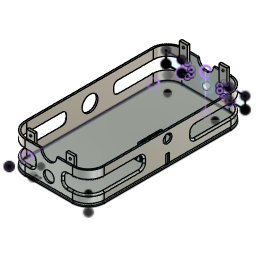
enclosure_bottom (Autodesk Fusion 360 design; units mm, degrees)
Autodesk Fusion 360 part; units mm, degrees
sketch "Sketch1" plane through (0, 0, 0) normal (0, 0, 1) x (1, 0, 0)
  line L0 (20, 0) -> (80, 0)
  line L1 (100, 20) -> (100, 180)
  line L2 (80, 200) -> (20, 200)
  line L3 (0, 180) -> (0, 20)
  arc A0 (0, 20) -> (20, 0) centre (20, 20) ccw
  arc A1 (80, 0) -> (100, 20) centre (80, 20) ccw
  arc A2 (100, 180) -> (80, 200) centre (80, 180) ccw
  arc A3 (20, 200) -> (0, 180) centre (20, 180) ccw
  line L4 (20, 2) -> (80, 2)
  arc A4 (80, 2) -> (98, 20) centre (80, 20) ccw
  line L5 (98, 20) -> (98, 180)
  arc A5 (98, 180) -> (80, 198) centre (80, 180) ccw
  line L6 (80, 198) -> (20, 198)
  arc A6 (20, 198) -> (2, 180) centre (20, 180) ccw
  line L7 (2, 180) -> (2, 20)
  arc A7 (2, 20) -> (20, 2) centre (20, 20) ccw
  point P0 (100, 0)
  point P1 (0, 200)
  dimension "d1" = 100
  dimension "d2" = 200
  dimension "d3" = 20
  dimension "d4" = -2
  constraint horizontal L0
  constraint vertical L1
  constraint horizontal L2
  constraint vertical L3
  constraint coincident origin L0
  constraint coincident origin L3
  constraint tangent L0 A0
  constraint tangent L3 A0
  constraint coincident P0 L0
  constraint coincident P0 L1
  constraint tangent L0 A1
  constraint tangent L1 A1
  constraint equal A0 A1
  constraint tangent L1 A2
  constraint tangent L2 A2
  constraint equal A0 A2
  constraint coincident P1 L2
  constraint coincident P1 L3
  constraint tangent L2 A3
  constraint tangent L3 A3
  constraint equal A0 A3
  measures "d1" distance of origin P0
  measures "d2" distance of origin P1
  measures "d3" radius of A0
extrude "Extrude1" add sketch "Sketch1" along normal blind 1.5 contours L4 A4 L5 A5 L6 A6 L7 A7
extrude "Extrude2" add sketch "Sketch1" along normal blind 40
sketch "Sketch2" plane through (0, 0, 0) normal (0, -1, 0) x (1, 0, 0)
  line L0 (20, 0) -> (80, 0)
  line L1 (80, 0) -> (80, 40)
  line L2 (80, 40) -> (20, 40)
  line L3 (20, 40) -> (20, 0)
  circle A0 centre (50, 40) radius 10
  dimension "d9" = 20
  constraint midpoint L2 A0.centre
  measures "d9" diameter of A0
sketch "Sketch3" plane through (0, 200, 0) normal (0, 1, 0) x (-1, 0, 0)
  line L0 (-80, 0) -> (-20, 0)
  line L1 (-20, 0) -> (-20, 40)
  line L2 (-20, 40) -> (-80, 40)
  line L3 (-80, 40) -> (-80, 0)
  circle A0 centre (-50, 40) radius 10
  dimension "d10" = 20
  constraint midpoint L2 A0.centre
  measures "d10" diameter of A0
extrude "Extrude3" cut sketch "Sketch3" against normal blind 10 contours L2 A0 picked at (-47.135, 36.6429)
extrude "Extrude4" cut sketch "Sketch2" against normal blind 10 contours L2 A0 picked at (52.865, 36.6429)
sketch "Sketch4" plane through (0, 0, 0) normal (-1, 0, 0) x (0, -1, 0)
  line L0 (-180, 0) -> (-20, 0)
  line L1 (-20, 0) -> (-20, 40)
  line L2 (-20, 40) -> (-180, 40)
  line L3 (-180, 40) -> (-180, 0)
  line L4 (-179.9999, 28) -> (-134.9999, 28)
  line L5 (-129.9999, 23) -> (-129.9999, 18)
  line L6 (-134.9999, 13) -> (-179.9999, 13)
  line L7 (-179.9999, 13) -> (-179.9999, 28)
  line L8 (-100, 40) -> (-100, 0) construction
  line L9 (-65.0001, 13) -> (-20.0001, 13)
  line L10 (-70.0001, 23) -> (-70.0001, 18)
  line L11 (-20.0001, 28) -> (-65.0001, 28)
  line L12 (-20.0001, 13) -> (-20.0001, 28)
  arc A0 (-129.9999, 23) -> (-134.9999, 28) centre (-134.9999, 23) ccw
  arc A1 (-134.9999, 13) -> (-129.9999, 18) centre (-134.9999, 18) ccw
  arc A2 (-65.0001, 28) -> (-70.0001, 23) centre (-65.0001, 23) ccw
  arc A3 (-70.0001, 18) -> (-65.0001, 13) centre (-65.0001, 18) ccw
  line L13 (-179.9999, 13) -> (-219.9999, 13)
  line L14 (-219.9999, 13) -> (-219.9999, 28)
  line L15 (-219.9999, 28) -> (-179.9999, 28)
  line L16 (-179.9999, 28) -> (-179.9999, 13)
  circle A4 centre (-100, 20) radius 10
  point P0 (-129.9999, 28)
  dimension "d15" = 50
  dimension "d16" = 15
  dimension "d17" = 0.0001
  dimension "d18" = 12
  dimension "d24" = 5
  dimension "d57" = 40
  dimension "d58" = 15
  dimension "d124" = 20
  dimension "d139" = 20
  constraint horizontal L4
  constraint vertical L5
  constraint horizontal L6
  constraint vertical L7
  constraint midpoint L2 L8.start
  constraint perpendicular L2 L8
  constraint symmetric L4.start L8 L11.start
  constraint symmetric L6.end L8 L9.end
  constraint coincident P0 L4
  constraint coincident P0 L5
  constraint tangent L4 A0
  constraint tangent L5 A0
  constraint tangent L5 A1
  constraint tangent L6 A1
  constraint equal A0 A1
  constraint tangent L10 A2
  constraint tangent L11 A2
  constraint equal A0 A2
  constraint tangent L9 A3
  constraint tangent L10 A3
  constraint equal A0 A3
  constraint horizontal L13
  constraint vertical L14
  constraint horizontal L15
  constraint vertical L16
  constraint midpoint L8 A4.centre
  measures "d15" distance of L4.start P0
  measures "d16" distance of L4.start L6.end
  measures "d17" distance of L3 L7
  measures "d18" distance of L2 L4
  measures "d24" radius of A0
  measures "d57" distance of L6.end L13.end
  measures "d58" distance of L6.end L4.start
  measures "d124" diameter of A4
  measures "d139" distance of L2 A4.centre
sketch "Sketch5" plane through (0, 0, 0) normal (0, -1, 0) x (1, 0, 0)
  arc A0 (40, 40) -> (60, 40) centre (50, 40) ccw
  line L0 (40, 40) -> (20, 40)
  line L1 (20, 40) -> (20, 0)
  line L2 (20, 0) -> (80, 0)
  line L3 (80, 0) -> (80, 40)
  line L4 (80, 40) -> (60, 40)
  line L5 (20, 28) -> (27, 28)
  line L6 (32, 23) -> (32, 18)
  line L7 (27, 13) -> (20, 13)
  line L8 (20, 13) -> (20, 28)
  line L9 (50, 30) -> (50, -15.7187) construction
  line L10 (50, 30) -> (50, -15.7187) construction
  line L11 (73, 13) -> (80, 13)
  line L12 (68, 23) -> (68, 18)
  line L13 (80, 28) -> (73, 28)
  line L14 (80, 13) -> (80, 28)
  line L15 (20, 28) -> (0, 28)
  line L16 (0, 28) -> (0, 13)
  line L17 (0, 13) -> (20, 13)
  line L18 (20, 13) -> (20, 28)
  line L19 (100, 13) -> (80, 13)
  line L20 (100, 28) -> (100, 13)
  line L21 (80, 28) -> (100, 28)
  line L22 (80, 13) -> (80, 28)
  arc A1 (32, 23) -> (27, 28) centre (27, 23) ccw
  arc A2 (27, 13) -> (32, 18) centre (27, 18) ccw
  arc A3 (68, 18) -> (73, 13) centre (73, 18) ccw
  arc A4 (73, 28) -> (68, 23) centre (73, 23) ccw
  arc A5 (20, 28) -> (20, 13) centre (20, 20.5) ccw
  line L23 (20, 13) -> (2, 13)
  line L24 (2, 28) -> (20, 28)
  circle A6 centre (50, 13.9414) radius 6.75
  point P0 (32, 28)
  dimension "d19" = 12
  dimension "d20" = 15
  dimension "d21" = 12
  dimension "d22" = 20
  dimension "d23" = 15
  dimension "d25" = 5
  dimension "d54" = 18
  dimension "d140" = 13.5
  constraint horizontal L5
  constraint vertical L6
  constraint horizontal L7
  constraint vertical L8
  constraint coincident L1 L5.start
  constraint midpoint A0 L9.start
  constraint vertical L9
  constraint symmetric L5.start L9 L13.start
  constraint symmetric L7.end L9 L11.end
  constraint symmetric L10.start L9 L9.start
  constraint symmetric L10.end L9 L9.end
  constraint horizontal L15
  constraint vertical L16
  constraint horizontal L17
  constraint vertical L18
  constraint symmetric L9 L15.end L20.start
  constraint symmetric L9 L16.end L19.start
  constraint symmetric L9 L7.end L11.end
  constraint coincident P0 L5
  constraint coincident P0 L6
  constraint tangent L5 A1
  constraint tangent L6 A1
  constraint tangent L6 A2
  constraint tangent L7 A2
  constraint equal A1 A2
  constraint tangent L11 A3
  constraint tangent L12 A3
  constraint equal A1 A3
  constraint tangent L12 A4
  constraint tangent L13 A4
  constraint equal A1 A4
  constraint tangent L5 A5
  constraint coincident L17 L23.end
  constraint coincident L15 L24.start
  constraint tangent A5 L24
  constraint coincident L9 A6.centre
  measures "d19" distance of L5.start P0
  measures "d20" distance of L5.start L7.end
  measures "d21" distance of L0 L5
  measures "d22" distance of L5.start L15.end
  measures "d23" distance of L5.start L7.end
  measures "d25" radius of A1
  measures "d54" distance of L7.end L23.end
  measures "d140" diameter of A6
extrude "Extrude5" cut sketch "Sketch5" against normal blind 21 contours L1 L5 L6 L7 L8 L18 A1 A2 | L15 L16 L17 A5 L23 L24 | L1 L8 L18 A5
extrude "Extrude6" cut sketch "Sketch4" against normal blind 10 contours L1 L9 L10 L11 L12 A2 A3
ref_plane "WorkPlane1" through (0, 100, 0) normal (0, 1, 0) x (0, 0, 1)
ref_plane "WorkPlane2" through (50, 0, 0) normal (1, 0, 0) x (0, 1, 0)
extrude "Extrude7" cut sketch "Sketch4" against normal blind 10 contours L3 L4 L5 L6 L7 A0 A1 L16
extrude "Extrude8" cut sketch "Sketch5" against normal blind 21 contours L3 L14 L19 L20 L21 L22 | L3 L11 L12 L13 L14 L22 A3 A4
sketch "Sketch6" plane through (0, 198, 0) normal (0, -1, 0) x (1, 0, 0)
  arc A0 (40, 40) -> (60, 40) centre (50, 40) ccw
  line L0 (40, 40) -> (20, 40)
  line L1 (20, 40) -> (20, 1.5)
  line L2 (20, 1.5) -> (80, 1.5)
  line L3 (80, 1.5) -> (80, 40)
  line L4 (80, 40) -> (60, 40)
  line L5 (80, 28) -> (100, 28)
  line L6 (80, 28) -> (73, 28)
  arc A1 (73, 28) -> (68, 23) centre (73, 23) ccw
  line L7 (68, 23) -> (68, 18)
  arc A2 (68, 18) -> (73, 13) centre (73, 18) ccw
  line L8 (73, 13) -> (80, 13)
  line L9 (100, 13) -> (80, 13)
  line L10 (32, 23) -> (32, 18)
  arc A3 (32, 23) -> (27, 28) centre (27, 23) ccw
  line L11 (20, 28) -> (27, 28)
  line L12 (20, 28) -> (0, 28)
  arc A4 (27, 13) -> (32, 18) centre (27, 18) ccw
  line L13 (27, 13) -> (20, 13)
  line L14 (0, 13) -> (20, 13)
  line L15 (0, 28) -> (0, 13)
  line L16 (100, 28) -> (100, 13)
  line L17 (0, 28) -> (0, 13)
  line L18 (100, 28) -> (80, 28)
  line L19 (80, 28) -> (80, 13)
  line L20 (80, 13) -> (100, 13)
  line L21 (20, 28) -> (0, 28)
  line L22 (0, 13) -> (20, 13)
  line L23 (50, 30) -> (50, -15.7187)
  line L24 (20, 13) -> (0, 13)
  line L25 (0, 28) -> (0, 13)
  line L26 (0, 28) -> (20, 28)
  line L27 (20, 28) -> (20, 13)
  constraint coincident L12.end L15.start
  constraint coincident L14.start L15.end
  constraint coincident L5.end L16.start
  constraint coincident L9.start L16.end
  constraint coincident L5.start L6.start
  constraint coincident L8.end L9.end
  constraint coincident L11.start L12.start
  constraint coincident L13.end L14.end
  constraint symmetric L5.end L23 L12.end
  constraint symmetric L9.start L23 L14.start
  constraint symmetric L5.start L23 L11.start
  constraint symmetric L8.end L23 L13.end
extrude "Extrude13" cut sketch "Sketch6" along normal blind 21 contours L3 L5 L9 L16 L18 L19 L20
sketch "Sketch7" plane through (100, 0, 0) normal (1, 0, 0) x (0, 1, 0)
  line L0 (20, 28) -> (21, 28)
  line L1 (21, 28) -> (21, 13)
  line L2 (21, 13) -> (20, 13)
  line L3 (20, 13) -> (20, 0)
  line L4 (20, 0) -> (180, 0)
  line L5 (180, 28) -> (180, 40)
  line L6 (180, 40) -> (20, 40)
  line L7 (20, 40) -> (20, 28)
  line L8 (20.0001, 28) -> (65.0001, 28)
  arc A0 (70.0001, 23) -> (65.0001, 28) centre (65.0001, 23) ccw
  line L9 (70.0001, 23) -> (70.0001, 18)
  arc A1 (65.0001, 13) -> (70.0001, 18) centre (65.0001, 18) ccw
  line L10 (65.0001, 13) -> (20.0001, 13)
  line L11 (179.9999, 28) -> (134.9999, 28)
  arc A2 (134.9999, 28) -> (129.9999, 23) centre (134.9999, 23) ccw
  line L12 (129.9999, 23) -> (129.9999, 18)
  arc A3 (129.9999, 18) -> (134.9999, 13) centre (134.9999, 18) ccw
  line L13 (134.9999, 13) -> (179.9999, 13)
  arc A4 (20.0001, 28) -> (20.0001, 13) centre (20.0001, 20.5) ccw
  line L14 (179.9999, 28) -> (179.9999, 13)
  line L15 (177, 28) -> (180, 28)
  line L16 (180, 0) -> (180, 13)
  line L17 (180, 13) -> (177, 13)
  line L18 (177, 13) -> (177, 28)
  constraint coincident L10.end A4.end
  constraint coincident L8.start A4.start
  constraint tangent L8 A4
  constraint coincident L11.start L14.start
  constraint coincident L13.end L14.end
extrude "Extrude11" cut sketch "Sketch7" against normal blind 10 contours L1 L8 A0 L9 A1 L10 | L11 L13 L14 L15 L17 L18 | L11 A2 L12 A3 L13 L18
extrude "Extrude12" cut sketch "Sketch6" against normal blind 21 contours L3 L5 L9 L16 L18 L19 L20
extrude "Extrude14" cut sketch "Sketch5" against normal blind 1000 contours L1 L5 L6 L7 L8 L18 A1 A2
extrude "Extrude15" cut sketch "Sketch5" against normal blind 1000 contours L3 L11 L12 L13 L14 L22 A3 A4
extrude "Extrude16" cut sketch "Sketch6" along normal blind 10 contours L1 L12 L14 L15 L17 L21 L22 L24 L25 L26 L27
extrude "Extrude17" cut sketch "Sketch6" along normal blind 21 contours L1 L12 L14 L15 L17 L21 L22 L24 L25 L26 L27
extrude "Extrude18" cut sketch "Sketch4" against normal blind 21 contours L3 L7 L13 L14 L15 L16
sketch "Sketch8" plane through (100, 0, 0) normal (1, 0, 0) x (0, 1, 0)
  line L0 (134.9999, 28) -> (180, 28)
  line L1 (180, 28) -> (180, 40)
  line L2 (180, 40) -> (20, 40)
  line L3 (20, 40) -> (20, 28)
  line L4 (20, 28) -> (65.0001, 28)
  arc A0 (70.0001, 23) -> (65.0001, 28) centre (65.0001, 23) ccw
  line L5 (70.0001, 23) -> (70.0001, 18)
  arc A1 (65.0001, 13) -> (70.0001, 18) centre (65.0001, 18) ccw
  line L6 (65.0001, 13) -> (20, 13)
  line L7 (20, 13) -> (20, 0)
  line L8 (20, 0) -> (180, 0)
  line L9 (180, 0) -> (180, 13)
  line L10 (180, 13) -> (134.9999, 13)
  arc A2 (129.9999, 18) -> (134.9999, 13) centre (134.9999, 18) ccw
  line L11 (129.9999, 18) -> (129.9999, 23)
  arc A3 (134.9999, 28) -> (129.9999, 23) centre (134.9999, 23) ccw
  circle A4 centre (100, 23.2658) radius 5.55
  dimension "d127" = 11.1
  measures "d127" diameter of A4
sketch "Sketch9" plane through (98, 0, 0) normal (-1, 0, 0) x (0, -1, 0)
  line L0 (-180, 28) -> (-134.9999, 28)
  arc A0 (-129.9999, 23) -> (-134.9999, 28) centre (-134.9999, 23) ccw
  line L1 (-129.9999, 23) -> (-129.9999, 18)
  arc A1 (-134.9999, 13) -> (-129.9999, 18) centre (-134.9999, 18) ccw
  line L2 (-134.9999, 13) -> (-180, 13)
  line L3 (-180, 13) -> (-180, 1.5)
  line L4 (-180, 1.5) -> (-20, 1.5)
  line L5 (-20, 1.5) -> (-20, 13)
  line L6 (-20, 13) -> (-65.0001, 13)
  arc A2 (-70.0001, 18) -> (-65.0001, 13) centre (-65.0001, 18) ccw
  line L7 (-70.0001, 18) -> (-70.0001, 23)
  arc A3 (-65.0001, 28) -> (-70.0001, 23) centre (-65.0001, 23) ccw
  line L8 (-65.0001, 28) -> (-20, 28)
  line L9 (-20, 28) -> (-20, 40)
  line L10 (-20, 40) -> (-180, 40)
  line L11 (-180, 40) -> (-180, 28)
  line L12 (-101.25, 1.5) -> (-98.75, 1.5)
  line L13 (-98.75, 1.5) -> (-98.75, 13.5)
  line L14 (-98.75, 13.5) -> (-101.25, 13.5)
  line L15 (-101.25, 13.5) -> (-101.25, 1.5)
  line L16 (-100, 40) -> (-100, 0)
  dimension "d68" = 2.5
  dimension "d69" = 12
  dimension "d70" = 1.25
  constraint horizontal L12
  constraint vertical L13
  constraint horizontal L14
  constraint vertical L15
  constraint coincident L4 L12.start
  measures "d68" distance of L12.start L12.end
  measures "d69" distance of L12.start L14.end
  measures "d70" distance of L15 L16
extrude "Extrude20" cut sketch "Sketch9" against normal blind 10 contours L4 L12 L14 L15 L16 | L4 L12 L13 L14 L16
fillet "Fillet1" radius 1 3 edges at (100, 101.25, 7.5) (100, 100, 13.5) (100, 98.75, 7.5)
sketch "Sketch10" plane through (0, 0, 1.5) normal (0, 0, 1) x (-1, 0, 0)
  arc A0 (-2, -20) -> (-20, -2) centre (-20, -20) ccw
  line L0 (-20, -2) -> (-80, -2)
  arc A1 (-80, -2) -> (-98, -20) centre (-80, -20) ccw
  line L1 (-98, -20) -> (-98, -98.75)
  line L2 (-98, -98.75) -> (-99, -98.75)
  arc A2 (-100, -97.75) -> (-99, -98.75) centre (-99, -97.75) ccw
  line L3 (-100, -97.75) -> (-100, -102.25)
  arc A3 (-99, -101.25) -> (-100, -102.25) centre (-99, -102.25) ccw
  line L4 (-99, -101.25) -> (-98, -101.25)
  line L5 (-98, -101.25) -> (-98, -180)
  arc A4 (-98, -180) -> (-80, -198) centre (-80, -180) ccw
  line L6 (-80, -198) -> (-20, -198)
  arc A5 (-20, -198) -> (-2, -180) centre (-20, -180) ccw
  line L7 (-2, -180) -> (-2, -20)
  line L8 (-98, -98.75) -> (-98, -87.3313)
  line L9 (-98, -98.75) -> (-98, -88.6307)
  line L10 (-98, -98.75) -> (-98, -89.4428)
  line L11 (-98, -98.75) -> (-98, -92.2096)
  line L12 (-98, -98.75) -> (-98, -86.75)
  line L13 (-98, -87.3313) -> (-78, -87.3313)
  line L14 (-78, -87.3313) -> (-78, -113.8313)
  line L15 (-78, -113.8313) -> (-98, -113.8313)
  line L16 (-99.5, -98.75) -> (-99.5, -85.8313)
  line L17 (-99.5, -85.8313) -> (-76.5, -85.8313)
  line L18 (-76.5, -85.8313) -> (-76.5, -115.3313)
  line L19 (-76.5, -115.3313) -> (-98, -115.3313)
  dimension "d77" = 12
  dimension "d78" = 20
  dimension "d79" = 26.5
  dimension "d80" = -1.5
  constraint coincident L1.end L2.start
  constraint coincident L1 L8.end
  constraint perpendicular L2 L8
  constraint coincident L8 L9.end
  constraint coincident L8 L10.end
  constraint coincident L8 L11.end
  constraint parallel L8 L12
  constraint perpendicular L8 L13
  constraint perpendicular L13 L14
  constraint coincident L5 L15.end
  constraint perpendicular L5 L15
  measures "d77" distance of L1.end L12.end
  measures "d78" distance of L8.end L13.end
  measures "d79" distance of L13.end L14.end
extrude "Extrude21" add sketch "Sketch10" along normal blind 20 contours L1 L5 L12 L13 L14 L15 L17 L18 L19
sketch "Sketch11" plane through (0, 87.3313, 0) normal (0, 1, 0) x (-1, 0, 0)
  line L0 (-98, 1.5) -> (-78, 1.5)
  line L1 (-78, 1.5) -> (-78, 21.5)
  line L2 (-78, 21.5) -> (-98, 21.5)
  line L3 (-98, 21.5) -> (-98, 1.5)
  circle A0 centre (-90.3989, 7.5) radius 4
  dimension "d83" = 8
  dimension "d84" = 6
  measures "d83" diameter of A0
  measures "d84" distance of L0 A0.centre
extrude "Extrude22" cut sketch "Sketch11" against normal blind 1 contours A0
sketch "Sketch12" plane through (0, 113.8313, 0) normal (0, -1, 0) x (1, 0, 0)
  line L0 (78, 1.5) -> (98, 1.5)
  line L1 (98, 1.5) -> (98, 21.5)
  line L2 (98, 21.5) -> (78, 21.5)
  line L3 (78, 21.5) -> (78, 1.5)
  circle A0 centre (88, 7.5) radius 4
  dimension "d87" = 8
  dimension "d88" = 6
  measures "d87" diameter of A0
  measures "d88" distance of L0 A0.centre
extrude "Extrude23" cut sketch "Sketch12" against normal blind 1 contours A0
sketch "Sketch13" plane through (0, 85.8313, 0) normal (0, -1, 0) x (1, 0, 0)
  line L0 (76.5, 1.5) -> (98, 1.5)
  line L1 (98, 1.5) -> (98, 21.5)
  line L2 (98, 21.5) -> (76.5, 21.5)
  line L3 (76.5, 21.5) -> (76.5, 1.5)
  circle A0 centre (80.5, 17.4329) radius 2
  dimension "d91" = 4
  dimension "d92" = 4
  measures "d91" diameter of A0
  measures "d92" distance of L3 A0.centre
extrude "Extrude24" cut sketch "Sketch13" against normal blind 10 contours A0
sketch "Sketch14" plane through (0, 115.3313, 0) normal (0, 1, 0) x (-1, 0, 0)
  line L0 (-98, 1.5) -> (-76.5, 1.5)
  line L1 (-76.5, 1.5) -> (-76.5, 21.5)
  line L2 (-76.5, 21.5) -> (-98, 21.5)
  line L3 (-98, 21.5) -> (-98, 1.5)
  circle A0 centre (-81.838, 17.5) radius 2
  dimension "d95" = 4
  dimension "d96" = 4
  measures "d95" diameter of A0
  measures "d96" distance of L2 A0.centre
extrude "Extrude25" cut sketch "Sketch14" against normal blind 4 contours A0
fillet "Fillet2" radius 2 12 edges at (76.5, 0, 13) (69.4645, 0, 14.4645) (68, 0, 20.5) (69.4645, 0, 26.5355) (76.5, 0, 28) (94.1421, 5.8579, 28) (100, 42.5001, 28) (100, 68.5356, 26.5355) (100, 70.0001, 20.5) (100, 68.5356, 14.4645) (100, 42.5001, 13) (94.1421, 5.8579, 13)
fillet "Fillet3" radius 2 12 edges at (100, 129.9999, 20.5) (100, 131.4644, 26.5355) (100, 157.4999, 28) (94.1421, 194.1421, 28) (76.5, 200, 28) (69.4645, 200, 26.5355) (68, 200, 20.5) (69.4645, 200, 14.4645) (76.5, 200, 13) (94.1421, 194.1421, 13) (100, 157.4999, 13) (100, 131.4644, 14.4645)
fillet "Fillet4" radius 2 12 edges at (0, 70.0001, 20.5) (0, 68.5356, 26.5355) (0, 42.5001, 28) (5.8579, 5.8579, 28) (23.5, 0, 28) (30.5355, 0, 26.5355) (32, 0, 20.5) (30.5355, 0, 14.4645) (23.5, 0, 13) (5.8579, 5.8579, 13) (0, 42.5001, 13) (0, 68.5356, 14.4645)
fillet "Fillet5" radius 2 12 edges at (30.5355, 200, 14.4645) (32, 200, 20.5) (30.5355, 200, 26.5355) (23.5, 200, 28) (5.8579, 194.1421, 28) (0, 157.4999, 28) (0, 131.4644, 26.5355) (0, 129.9999, 20.5) (0, 131.4644, 14.4645) (0, 157.4999, 13) (5.8579, 194.1421, 13) (23.5, 200, 13)
sketch "Sketch15" plane through (0, 0, 1.5) normal (0, 0, 1) x (-1, 0, 0)
  line L0 (-76.5, -115.3313) -> (-98, -115.3313)
  line L1 (-98, -115.3313) -> (-98, -180)
  arc A0 (-98, -180) -> (-80, -198) centre (-80, -180) ccw
  line L2 (-80, -198) -> (-20, -198)
  arc A1 (-20, -198) -> (-2, -180) centre (-20, -180) ccw
  line L3 (-2, -180) -> (-2, -20)
  arc A2 (-2, -20) -> (-20, -2) centre (-20, -20) ccw
  line L4 (-20, -2) -> (-80, -2)
  arc A3 (-80, -2) -> (-98, -20) centre (-80, -20) ccw
  line L5 (-98, -20) -> (-98, -85.8313)
  line L6 (-98, -85.8313) -> (-76.5, -85.8313)
  line L7 (-76.5, -85.8313) -> (-76.5, -115.3313)
  line L8 (-28, -2) -> (-34, -2)
  line L9 (-34, -2) -> (-34, -6)
  line L10 (-34, -6) -> (-28, -6)
  line L11 (-28, -6) -> (-28, -2)
  line L12 (-2, -180) -> (-2, -20)
  dimension "d109" = 6
  dimension "d110" = 4
  dimension "d111" = 26
  constraint horizontal L8
  constraint vertical L9
  constraint horizontal L10
  constraint vertical L11
  constraint coincident L4 L8.start
  measures "d109" distance of L8.start L8.end
  measures "d110" distance of L8.start L10.end
  measures "d111" distance of L11 L12
fillet "Fillet7" radius 3.5 8 edges at (50, 200, 0) (5.8579, 194.1421, 0) (0, 100, 0) (5.8579, 5.8579, 0) (50, 0, 0) (94.1421, 5.8579, 0) (100, 100, 0) (94.1421, 194.1421, 0)
sketch "Sketch16" plane through (0, 0, 40) normal (0, 0, 1) x (-1, 0, 0)
  line L0 (-60, -2) -> (-60, 0)
  line L1 (-60, 0) -> (-80, 0)
  arc A0 (-80, 0) -> (-100, -20) centre (-80, -20) ccw
  line L2 (-100, -20) -> (-100, -180)
  arc A1 (-100, -180) -> (-80, -200) centre (-80, -180) ccw
  line L3 (-80, -200) -> (-60, -200)
  line L4 (-60, -200) -> (-60, -198)
  line L5 (-60, -198) -> (-80, -198)
  arc A2 (-98, -180) -> (-80, -198) centre (-80, -180) ccw
  line L6 (-98, -180) -> (-98, -20)
  arc A3 (-80, -2) -> (-98, -20) centre (-80, -20) ccw
  line L7 (-80, -2) -> (-60, -2)
  line L8 (-70, -2) -> (-80, -2)
  line L9 (-80, -2) -> (-80, -5)
  line L10 (-80, -5) -> (-70, -5)
  line L11 (-70, -5) -> (-70, -2)
  line L12 (-30, -2) -> (-20, -2)
  line L13 (-20, -2) -> (-20, -5)
  line L14 (-20, -5) -> (-30, -5)
  line L15 (-30, -5) -> (-30, -2)
  line L16 (-40, 0) -> (-40, -2)
  dimension "d114" = 10
  dimension "d115" = 3
  dimension "d116" = 10
  dimension "d117" = 10
  dimension "d118" = 3
  dimension "d119" = 10
  constraint horizontal L8
  constraint vertical L9
  constraint horizontal L10
  constraint vertical L11
  constraint coincident L7 L8.start
  constraint horizontal L12
  constraint vertical L13
  constraint horizontal L14
  constraint vertical L15
  measures "d114" distance of L8.start A3.start
  measures "d115" distance of L8.start L10.end
  measures "d116" distance of L0 L11
  measures "d117" distance of L12.start L12.end
  measures "d118" distance of L12.start L14.end
  measures "d119" distance of L15 L16
extrude "Extrude26" add sketch "Sketch16" along normal mid plane 20 contours L7 L8 L9 L10 L11 | L12 L13 L14 L15
mirror "Mirror2" about plane through (0, 100, 0) normal (0, 1, 0) of "Extrude26"
extrude "Extrude27" cut sketch "Sketch4" against normal blind 10 contours A4
sketch "Sketch17" plane through (100, 0, 0) normal (1, 0, 0) x (0, 1, 0)
  line L0 (20, 3.5) -> (97.75, 3.5)
  line L1 (97.75, 3.5) -> (97.75, 14.5)
  line L2 (97.75, 14.5) -> (102.25, 14.5)
  line L3 (102.25, 14.5) -> (102.25, 3.5)
  line L4 (102.25, 3.5) -> (180, 3.5)
  line L5 (180, 3.5) -> (180, 11)
  line L6 (180, 11) -> (134.9999, 11)
  arc A0 (127.9999, 18) -> (134.9999, 11) centre (134.9999, 18) ccw
  line L7 (127.9999, 18) -> (127.9999, 23)
  arc A1 (134.9999, 30) -> (127.9999, 23) centre (134.9999, 23) ccw
  line L8 (134.9999, 30) -> (180, 30)
  line L9 (180, 30) -> (180, 40)
  line L10 (180, 40) -> (20, 40)
  line L11 (20, 40) -> (20, 30)
  line L12 (20, 30) -> (65.0001, 30)
  arc A2 (72.0001, 23) -> (65.0001, 30) centre (65.0001, 23) ccw
  line L13 (72.0001, 23) -> (72.0001, 18)
  arc A3 (65.0001, 11) -> (72.0001, 18) centre (65.0001, 18) ccw
  line L14 (65.0001, 11) -> (20, 11)
  line L15 (20, 11) -> (20, 3.5)
  circle A4 centre (100, 30.5728) radius 5.5
  dimension "d130" = 11
  measures "d130" diameter of A4
extrude "Extrude29" cut sketch "Sketch17" against normal blind 10 contours A4
sketch "Sketch18" plane through (98, 0, 0) normal (-1, 0, 0) x (0, -1, 0)
  circle A0 centre (-100, 30.5728) radius 5.5
  line L0 (-115.3313, 1.5) -> (-115.3313, 21.5)
  line L1 (-115.3313, 21.5) -> (-113.8313, 21.5)
  line L2 (-113.8313, 21.5) -> (-113.8313, 1.5)
  line L3 (-113.8313, 1.5) -> (-101.25, 1.5)
  line L4 (-101.25, 1.5) -> (-101.25, 13.5)
  line L5 (-101.25, 13.5) -> (-98.75, 13.5)
  line L6 (-98.75, 13.5) -> (-98.75, 1.5)
  line L7 (-98.75, 1.5) -> (-87.3313, 1.5)
  line L8 (-87.3313, 1.5) -> (-87.3313, 21.5)
  line L9 (-87.3313, 21.5) -> (-85.8313, 21.5)
  line L10 (-85.8313, 21.5) -> (-85.8313, 1.5)
  line L11 (-85.8313, 1.5) -> (-20, 1.5)
  line L12 (-20, 1.5) -> (-20, 13)
  line L13 (-20, 13) -> (-65.0001, 13)
  arc A1 (-70.0001, 18) -> (-65.0001, 13) centre (-65.0001, 18) ccw
  line L14 (-70.0001, 18) -> (-70.0001, 23)
  arc A2 (-65.0001, 28) -> (-70.0001, 23) centre (-65.0001, 23) ccw
  line L15 (-65.0001, 28) -> (-20, 28)
  line L16 (-20, 28) -> (-20, 40)
  line L17 (-20, 40) -> (-180, 40)
  line L18 (-180, 40) -> (-180, 28)
  line L19 (-180, 28) -> (-134.9999, 28)
  arc A3 (-129.9999, 23) -> (-134.9999, 28) centre (-134.9999, 23) ccw
  line L20 (-129.9999, 23) -> (-129.9999, 18)
  arc A4 (-134.9999, 13) -> (-129.9999, 18) centre (-134.9999, 18) ccw
  line L21 (-134.9999, 13) -> (-180, 13)
  line L22 (-180, 13) -> (-180, 1.5)
  line L23 (-180, 1.5) -> (-115.3313, 1.5)
  line L24 (-103.25, 1.5) -> (-103.25, 15.5)
  line L25 (-103.25, 15.5) -> (-96.75, 15.5)
  line L26 (-96.75, 15.5) -> (-96.75, 1.5)
  dimension "d133" = -2
extrude "Extrude30" add sketch "Sketch18" along normal blind 10 contours L3 L4 L5 L6 L7 L24 L25 L26
sketch "Sketch19" plane through (0, 200, 0) normal (0, 1, 0) x (-1, 0, 0)
  line L0 (-80, 3.5) -> (-20, 3.5)
  line L1 (-20, 3.5) -> (-20, 11)
  line L2 (-20, 11) -> (-27, 11)
  arc A0 (-34, 18) -> (-27, 11) centre (-27, 18) ccw
  line L3 (-34, 18) -> (-34, 23)
  arc A1 (-27, 30) -> (-34, 23) centre (-27, 23) ccw
  line L4 (-27, 30) -> (-20, 30)
  line L5 (-20, 30) -> (-20, 40)
  line L6 (-20, 40) -> (-40, 40)
  arc A2 (-60, 40) -> (-40, 40) centre (-50, 40) ccw
  line L7 (-60, 40) -> (-80, 40)
  line L8 (-80, 40) -> (-80, 30)
  line L9 (-80, 30) -> (-73, 30)
  arc A3 (-66, 23) -> (-73, 30) centre (-73, 23) ccw
  line L10 (-66, 23) -> (-66, 18)
  arc A4 (-73, 11) -> (-66, 18) centre (-73, 18) ccw
  line L11 (-73, 11) -> (-80, 11)
  line L12 (-80, 11) -> (-80, 3.5)
  circle A5 centre (-50, 13.4024) radius 6.8
  dimension "d136" = 13.6
  measures "d136" diameter of A5
extrude "Extrude32" cut sketch "Sketch5" against normal blind 10 contours A6
sketch "Sketch21" plane through (0, 2, 0) normal (0, -1, 0) x (1, 0, 0)
  line L0 (20, 40) -> (30, 40)
  line L1 (30, 40) -> (30, 50)
  line L2 (30, 50) -> (20, 50)
  line L3 (20, 50) -> (20, 40)
  circle A0 centre (25, 45) radius 1.4
  line L4 (50, 29.5494) -> (50, 1.0189)
  circle A1 centre (75, 45) radius 1.4
  dimension "d143" = 2.8
  dimension "d145" = 5
  dimension "d146" = 5
  constraint symmetric A0 L4 A1
  measures "d143" diameter of A0
  measures "d145" distance of L0 A0.centre
  measures "d146" distance of L1 A0.centre
extrude "Extrude33" cut sketch "Sketch21" against normal blind 1000 contours A0 | A1
sketch "Sketch22" plane through (0, 85.8313, 0) normal (0, -1, 0) x (1, 0, 0)
  circle A0 centre (80.5, 17.4329) radius 2
  line L0 (76.5, 1.5) -> (98, 1.5)
  line L1 (98, 1.5) -> (98, 21.5)
  line L2 (98, 21.5) -> (76.5, 21.5)
  line L3 (76.5, 21.5) -> (76.5, 1.5)
  line L4 (83.3082, 21.5) -> (79.3082, 21.5)
  line L5 (79.3082, 21.5) -> (79.3082, 1.5)
  line L6 (79.3082, 1.5) -> (83.3082, 1.5)
  line L7 (83.3082, 1.5) -> (83.3082, 21.5)
  dimension "d149" = 4
  dimension "d150" = 20
  constraint horizontal L4
  constraint vertical L5
  constraint horizontal L6
  constraint vertical L7
  constraint coincident L2 L4.start
  measures "d149" distance of L4.start L4.end
  measures "d150" distance of L4.start L6.end
extrude "Extrude34" cut sketch "Sketch22" against normal blind 50 contours A0 L0 L2 L4 L5 L6 L7
extrude "Extrude35" add 1 faces at (88.8835, 114.8313, 8.7709) along direction (0, -1, 0) blind 1
extrude "Extrude36" add 1 faces at (89.5155, 86.3313, 8.7709) along direction (0, 1, 0) blind 1
sketch "Sketch23" plane through (0, 115.3313, 0) normal (0, 1, 0) x (-1, 0, 0)
  line L0 (-79.3082, 15.8268) -> (-79.3082, 1.5)
  line L1 (-79.3082, 1.5) -> (-76.5, 1.5)
  line L2 (-76.5, 1.5) -> (-76.5, 21.5)
  line L3 (-76.5, 21.5) -> (-79.3082, 21.5)
  line L4 (-79.3082, 21.5) -> (-79.3082, 19.0391)
  arc A0 (-79.3082, 19.0391) -> (-81.0746, 19.3486) centre (-80.5, 17.4329) ccw
  arc A1 (-81.2633, 15.5843) -> (-81.0746, 19.3486) centre (-81.838, 17.5) ccw
  arc A2 (-81.2633, 15.5843) -> (-79.3082, 15.8268) centre (-80.5, 17.4329) ccw
  line L5 (-78.308, 21.5) -> (-81.808, 21.5)
  line L6 (-81.808, 21.5) -> (-81.808, 1.5)
  line L7 (-81.808, 1.5) -> (-78.308, 1.5)
  line L8 (-78.308, 1.5) -> (-78.308, 21.5)
  dimension "d157" = 3.5
  dimension "d158" = 20
  constraint horizontal L5
  constraint vertical L6
  constraint horizontal L7
  constraint vertical L8
  constraint coincident L3 L5.start
  measures "d157" distance of L5.start L5.end
  measures "d158" distance of L5.start L7.end
extrude "Extrude37" cut sketch "Sketch23" against normal blind 10 contours L0 L1 L3 L4 A0 A1 A2 L5 L7 L8
fillet "Fillet8" radius 5 1 edges at (76.5, 100.5813, 1.5)
